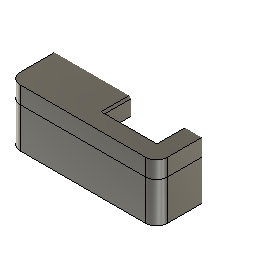
Password_key_ProMicro v1 (Autodesk Fusion 360 design; units mm, degrees)
Autodesk Fusion 360 part; units mm, degrees
sketch "Sketch1" plane through (0, 0, 0) normal (0, 0, 1) x (1, 0, 0)
  line L0 (0, 0) -> (33.5, 0)
  line L1 (33.5, 0) -> (33.5, 18.2)
  line L2 (33.5, 18.2) -> (0, 18.2)
  line L3 (0, 18.2) -> (0, 0)
  line L4 (-3, -3) -> (36.5, -3)
  line L5 (36.5, -3) -> (36.5, 21.2)
  line L6 (36.5, 21.2) -> (-3, 21.2)
  line L7 (-3, 21.2) -> (-3, -3)
  line L8 (0, 9.1) -> (-3, 9.1)
  line L9 (0, 12.85) -> (-3, 12.85)
  line L10 (-3, 12.85) -> (-3, 5.35)
  line L11 (-3, 5.35) -> (0, 5.35)
  line L12 (0, 5.35) -> (0, 12.85)
  line L13 (0, 12.85) -> (-3, 5.35) construction
  line L14 (-3, 12.85) -> (0, 5.35) construction
  circle A0 centre (0, 18.2) radius 0.5
  circle A1 centre (33.5, 18.2) radius 0.5
  circle A2 centre (0, 0) radius 0.5
  circle A3 centre (33.5, 0) radius 0.5
  point P0 (-1.5, 9.1)
  dimension "d1" = 33.5
  dimension "d2" = 18.2
  dimension "d3" = 3
  dimension "d4" = 7.5
  dimension "d10" = 1
  dimension "d11" = 1
  constraint horizontal L0
  constraint vertical L1
  constraint horizontal L2
  constraint vertical L3
  constraint coincident L0.start L3.end
  constraint midpoint L3 L8.start
  constraint midpoint L7 L8.end
  constraint horizontal L9
  constraint perpendicular L9 L10
  constraint parallel L9 L11
  constraint parallel L10 L12
  constraint coincident L13 P0
  constraint coincident L14 P0
  constraint coincident L3 L9.start
  constraint midpoint L8 P0
  constraint coincident L2.end L3.start
  constraint coincident L1.end L2.start
  constraint symmetric L8 A0 A2
  constraint symmetric L8 A1 A3
  measures "d1" distance of L0.start L0.end
  measures "d2" distance of L0.start L2.end
  measures "d4" distance of L9 L11
  measures "d10" diameter of A0
  measures "d11" diameter of A1
extrude "Extrude1" add sketch "Sketch1" against normal blind 1.75 contours L0 L1 L2 L3 L4 L5 L6 L7 L9 L11 A0 A1 A2 A3 makes body 1
extrude "Extrude2" add sketch "Sketch1" against normal blind 3 from surface at -1.75 bodies 1
fillet "Fillet1" radius 3 4 edges at (-3, -3, -2.375) (-3, 21.2, -2.375) (36.5, -3, -2.375) (36.5, 21.2, -2.375) on bodies 1
sketch "Sketch2" plane through (0, 0, 0) normal (0, 0, 1) x (1, 0, 0)
  line L0 (-3, 18.2) -> (-3, 12.85)
  line L1 (0, -3) -> (33.5, -3)
  line L2 (36.5, 0) -> (36.5, 18.2)
  line L3 (33.5, 21.2) -> (0, 21.2)
  line L4 (-3, 12.85) -> (0, 12.85)
  line L5 (0, 12.85) -> (0, 17.7)
  arc A0 (0.5, 18.2) -> (0, 17.7) centre (0, 18.2) ccw
  line L6 (0.5, 18.2) -> (33, 18.2)
  arc A1 (33.5, 17.7) -> (33, 18.2) centre (33.5, 18.2) ccw
  line L7 (33.5, 17.7) -> (33.5, 0.5)
  arc A2 (33, 0) -> (33.5, 0.5) centre (33.5, 0) ccw
  line L8 (33, 0) -> (0.5, 0)
  arc A3 (0, 0.5) -> (0.5, 0) centre (0, 0) ccw
  line L9 (0, 0.5) -> (0, 5.35)
  line L10 (0, 5.35) -> (-3, 5.35)
  arc A4 (36.5, 18.2) -> (33.5, 21.2) centre (33.5, 18.2) ccw
  arc A5 (0, 21.2) -> (-3, 18.2) centre (0, 18.2) ccw
  line L11 (-3, 5.35) -> (-3, 0)
  arc A6 (-3, 0) -> (0, -3) centre (0, 0) ccw
  arc A7 (33.5, -3) -> (36.5, 0) centre (33.5, 0) ccw
  line L12 (-1.4, 5.35) -> (-1.4, 0)
  arc A8 (-1.4, 0) -> (0, -1.4) centre (0, 0) ccw
  line L13 (0, -1.4) -> (33.5, -1.4)
  arc A9 (33.5, -1.4) -> (34.9, 0) centre (33.5, 0) ccw
  line L14 (34.9, 0) -> (34.9, 18.2)
  arc A10 (34.9, 18.2) -> (33.5, 19.6) centre (33.5, 18.2) ccw
  line L15 (33.5, 19.6) -> (0, 19.6)
  arc A11 (0, 19.6) -> (-1.4, 18.2) centre (0, 18.2) ccw
  line L16 (-1.4, 18.2) -> (-1.4, 12.85)
  dimension "d14" = -1.6
extrude "Extrude3" add sketch "Sketch2" along normal blind 6 contours L0 L1 L2 L3 L4 L10 A4 A5 L11 A6 A7 L12 A8 L13 A9 L14 A10 L15 A11 L16 bodies 1
sketch "Sketch3" plane through (0, 0, 6) normal (0, 0, 1) x (-1, 0, 0)
  line L0 (1.4, -5.35) -> (3, -5.35)
  line L1 (3, -5.35) -> (3, 0)
  arc A0 (3, 0) -> (0, 3) centre (0, 0) ccw
  line L2 (0, 3) -> (-33.5, 3)
  arc A1 (-33.5, 3) -> (-36.5, 0) centre (-33.5, 0) ccw
  line L3 (-36.5, 0) -> (-36.5, -18.2)
  arc A2 (-36.5, -18.2) -> (-33.5, -21.2) centre (-33.5, -18.2) ccw
  line L4 (-33.5, -21.2) -> (0, -21.2)
  arc A3 (0, -21.2) -> (3, -18.2) centre (0, -18.2) ccw
  line L5 (3, -18.2) -> (3, -12.85)
  line L6 (3, -12.85) -> (1.4, -12.85)
  line L7 (1.4, -12.85) -> (1.4, -18.2)
  arc A4 (0, -19.6) -> (1.4, -18.2) centre (0, -18.2) ccw
  line L8 (0, -19.6) -> (-33.5, -19.6)
  arc A5 (-34.9, -18.2) -> (-33.5, -19.6) centre (-33.5, -18.2) ccw
  line L9 (-34.9, -18.2) -> (-34.9, 0)
  arc A6 (-33.5, 1.4) -> (-34.9, 0) centre (-33.5, 0) ccw
  line L10 (-33.5, 1.4) -> (0, 1.4)
  arc A7 (1.4, 0) -> (0, 1.4) centre (0, 0) ccw
  line L11 (1.4, 0) -> (1.4, -5.35)
  arc A8 (-36.5, -18.2) -> (-33.5, -21.2) centre (-33.5, -18.2) ccw
  line L12 (-36.5, -18.2) -> (-36.5, 0)
  arc A9 (-33.5, 3) -> (-36.5, 0) centre (-33.5, 0) ccw
  line L13 (-33.5, 3) -> (0, 3)
  arc A10 (3, 0) -> (0, 3) centre (0, 0) ccw
  line L14 (3, 0) -> (3, -18.2)
  arc A11 (0, -21.2) -> (3, -18.2) centre (0, -18.2) ccw
  line L15 (0, -21.2) -> (-33.5, -21.2)
extrude "Extrude4" add sketch "Sketch3" 1 faces at (11.1667, -1.9333, 6) along normal blind 1.6 separate body contours L0 L6 L7 A4 L8 A5 L9 A6 L10 A7 L11 L14 on bodies 1 makes body 2
sketch "Sketch4" plane through (0, 0, 6) normal (0, 0, -1) x (1, 0, 0)
  line L0 (-3, 0) -> (-3, -18.2)
  arc A0 (-3, -18.2) -> (0, -21.2) centre (0, -18.2) ccw
  line L1 (0, -21.2) -> (33.5, -21.2)
  arc A1 (33.5, -21.2) -> (36.5, -18.2) centre (33.5, -18.2) ccw
  line L2 (36.5, -18.2) -> (36.5, 0)
  arc A2 (36.5, 0) -> (33.5, 3) centre (33.5, 0) ccw
  line L3 (33.5, 3) -> (0, 3)
  arc A3 (0, 3) -> (-3, 0) centre (0, 0) ccw
  line L4 (-3, -5.35) -> (0, -5.35)
  line L5 (0, -12.85) -> (-3, -12.85)
  line L6 (-3, -21.2) -> (-3, 3)
  line L7 (0, -5.35) -> (0, -12.85)
  line L8 (-3, -5.45) -> (0, -5.45)
  line L9 (-3, -9.1) -> (0, -9.1)
  line L10 (-3, -12.75) -> (0, -12.75)
  dimension "d19" = 0.1
  constraint midpoint L6 L9.start
  constraint midpoint L7 L9.end
  constraint symmetric L8.start L9 L10.start
  constraint symmetric L8.end L9 L10.end
extrude "Extrude5" add sketch "Sketch4" along normal blind 3 contours L0 L6 L7 L8 L9 | L0 L6 L7 L9 L10 bodies 2
sketch "Sketch5" plane through (0, 0, 6) normal (0, 0, -1) x (1, 0, 0)
  line L0 (0, -12.75) -> (-3, -12.75)
  line L1 (-3, -12.75) -> (-3, -18.2)
  arc A0 (-3, -18.2) -> (0, -21.2) centre (0, -18.2) ccw
  line L2 (0, -21.2) -> (33.5, -21.2)
  arc A1 (33.5, -21.2) -> (36.5, -18.2) centre (33.5, -18.2) ccw
  line L3 (36.5, -18.2) -> (36.5, 0)
  arc A2 (36.5, 0) -> (33.5, 3) centre (33.5, 0) ccw
  line L4 (33.5, 3) -> (0, 3)
  arc A3 (0, 3) -> (-3, 0) centre (0, 0) ccw
  line L5 (-3, 0) -> (-3, -5.45)
  line L6 (-3, -5.45) -> (0, -5.45)
  line L7 (0, -5.45) -> (0, -12.75)
  line L8 (-1.4, -5.35) -> (-3, -5.35)
  line L9 (-3, -5.35) -> (-3, 0)
  arc A4 (0, 3) -> (-3, 0) centre (0, 0) ccw
  line L10 (0, 3) -> (33.5, 3)
  arc A5 (36.5, 0) -> (33.5, 3) centre (33.5, 0) ccw
  line L11 (36.5, 0) -> (36.5, -18.2)
  arc A6 (33.5, -21.2) -> (36.5, -18.2) centre (33.5, -18.2) ccw
  line L12 (33.5, -21.2) -> (0, -21.2)
  arc A7 (-3, -18.2) -> (0, -21.2) centre (0, -18.2) ccw
  line L13 (-3, -18.2) -> (-3, -12.85)
  line L14 (-3, -12.85) -> (-1.4, -12.85)
  line L15 (-1.4, -12.85) -> (-1.4, -18.2)
  arc A8 (-1.4, -18.2) -> (0, -19.6) centre (0, -18.2) ccw
  line L16 (0, -19.6) -> (33.5, -19.6)
  arc A9 (33.5, -19.6) -> (34.9, -18.2) centre (33.5, -18.2) ccw
  line L17 (34.9, -18.2) -> (34.9, 0)
  arc A10 (34.9, 0) -> (33.5, 1.4) centre (33.5, 0) ccw
  line L18 (33.5, 1.4) -> (0, 1.4)
  arc A11 (0, 1.4) -> (-1.4, 0) centre (0, 0) ccw
  line L19 (-1.4, 0) -> (-1.4, -5.35)
  line L20 (-1.2, -12.85) -> (-1.2, -18.2)
  arc A12 (-1.2, -18.2) -> (0, -19.4) centre (0, -18.2) ccw
  line L21 (0, -19.4) -> (33.5, -19.4)
  arc A13 (33.5, -19.4) -> (34.7, -18.2) centre (33.5, -18.2) ccw
  line L22 (34.7, -18.2) -> (34.7, 0)
  arc A14 (34.7, 0) -> (33.5, 1.2) centre (33.5, 0) ccw
  line L23 (33.5, 1.2) -> (0, 1.2)
  arc A15 (0, 1.2) -> (-1.2, 0) centre (0, 0) ccw
  line L24 (-1.2, 0) -> (-1.2, -5.35)
  line L25 (-1.2, -12.85) -> (-1.2, -12.75)
  line L26 (-1.2, -12.75) -> (-1.2, -5.35)
  line L27 (0.4, -12.85) -> (0.4, -17.8)
  line L28 (0.4, -17.8) -> (33.1, -17.8)
  line L29 (33.1, -17.8) -> (33.1, -0.4)
  line L30 (33.1, -0.4) -> (0.4, -0.4)
  line L31 (0.4, -0.4) -> (0.4, -5.35)
  line L32 (0.4, -12.85) -> (0.4, -5.35)
  dimension "d22" = -0.2
  dimension "d23" = -1.8
  constraint coincident L0 L25.end
  constraint perpendicular L0 L25
  constraint perpendicular L8 L26
extrude "Extrude6" add sketch "Sketch5" along normal blind 3 contours L0 L6 L7 L20 A12 L21 A13 L22 A14 L23 A15 L24 L25 L26 bodies 2
sketch "Sketch6" plane through (0, 0, 7.6) normal (0, 0, 1) x (-1, 0, 0)
  line L0 (3, -18.2) -> (3, 0)
  arc A0 (3, 0) -> (0, 3) centre (0, 0) ccw
  line L1 (0, 3) -> (-33.5, 3)
  arc A1 (-33.5, 3) -> (-36.5, 0) centre (-33.5, 0) ccw
  line L2 (-36.5, 0) -> (-36.5, -18.2)
  arc A2 (-36.5, -18.2) -> (-33.5, -21.2) centre (-33.5, -18.2) ccw
  line L3 (-33.5, -21.2) -> (0, -21.2)
  arc A3 (0, -21.2) -> (3, -18.2) centre (0, -18.2) ccw
  line L4 (3, -9.1) -> (-36.5, -9.1)
  line L5 (-31.5, -16.09) -> (-17.52, -16.09)
  line L6 (-17.52, -16.09) -> (-17.52, -2.11)
  line L7 (-17.52, -2.11) -> (-31.5, -2.11)
  line L8 (-31.5, -2.11) -> (-31.5, -16.09)
  line L9 (-31.5, -16.09) -> (-17.52, -2.11) construction
  line L10 (-17.52, -16.09) -> (-31.5, -2.11) construction
  point P0 (-24.51, -9.1)
  dimension "d26" = 13.98
  dimension "d27" = 13.98
  dimension "d28" = 5
  constraint midpoint L0 L4.start
  constraint midpoint L2 L4.end
  constraint horizontal L5
  constraint perpendicular L5 L6
  constraint parallel L5 L7
  constraint parallel L6 L8
  constraint coincident L9 P0
  constraint coincident L10 P0
  constraint coincident L4 P0
  measures "d26" distance of L6.end L7.end
  measures "d27" distance of L5.end L6.end
  measures "d28" distance of L2 L8
extrude "Extrude7" add sketch "Sketch6" along normal blind 3 contours L0 L2 A2 L3 A3 L4 L5 L6 L8 | L0 A0 L1 A1 L2 L4 L6 L7 L8 bodies 2
extrude "Extrude8" cut 1 faces at (26.84, 6.77, 7.6) along direction (0, 0, -1) blind 2.947 on bodies 2 bodies 2
sketch "Sketch7" plane through (0, -1.2, 0) normal (0, -1, 0) x (1, 0, 0)
  line L0 (33.5, 6) -> (0, 6)
  line L1 (0, 6) -> (0, 3)
  line L2 (0, 3) -> (33.5, 3)
  line L3 (33.5, 3) -> (33.5, 6)
  line L4 (14.25, 3.4) -> (19.25, 3.4)
  line L5 (19.25, 3.4) -> (19.25, 5.2)
  line L6 (19.25, 5.2) -> (14.25, 5.2)
  line L7 (14.25, 5.2) -> (14.25, 3.4)
  line L8 (14.05, 3.2) -> (19.45, 3.2)
  line L9 (19.45, 3.2) -> (19.45, 5.4)
  line L10 (19.45, 5.4) -> (14.05, 5.4)
  line L11 (14.05, 5.4) -> (14.05, 3.2)
  line L12 (16.75, 3) -> (16.75, 6)
  line L13 (33.5, 6) -> (0, 6)
  point P0 (16.75, 5.4)
  dimension "d33" = 5
  dimension "d34" = 1.8
  dimension "d35" = 0.2
  dimension "d42" = 0.6
  constraint horizontal L4
  constraint vertical L5
  constraint horizontal L6
  constraint vertical L7
  constraint midpoint L2 L12.start
  constraint midpoint L0 L12.end
  constraint midpoint L10 P0
  constraint coincident L12 P0
  measures "d33" distance of L4.start L4.end
  measures "d34" distance of L4.start L6.end
  measures "d42" distance of L10 L13
extrude "Extrude9" add sketch "Sketch7" along normal blind 10 draft -45 contours L4 L6 L7 L12 | L4 L5 L6 L12 bodies 2
extrude "Extrude10" cut sketch "Sketch7" along normal blind 15 draft -45 from surface at 0.2 contours L4 L6 L7 L8 L10 L11 L12 | L4 L5 L6 L8 L9 L10 L12 | L4 L6 L7 L12 | L4 L5 L6 L12 bodies 1
ref_plane "WorkPlane1" through (16.75, 9.1, 0.625) normal (0, 1, 0) x (1, 0, 0)
mirror "Mirror1" about plane through (16.75, 9.1, 0.625) normal (0, 1, 0) of "Extrude9", "Extrude10"
sketch "Sketch8" plane through (34.7, 0, 0) normal (1, 0, 0) x (0, 1, 0)
  line L0 (18.2, 6) -> (0, 6)
  line L1 (0, 6) -> (0, 3)
  line L2 (0, 3) -> (18.2, 3)
  line L3 (18.2, 3) -> (18.2, 6)
  line L4 (9.1, 6) -> (9.1, 3)
  line L5 (11.6, 3.6) -> (6.6, 3.6)
  line L6 (6.6, 3.6) -> (6.6, 5.4)
  line L7 (6.6, 5.4) -> (11.6, 5.4)
  line L8 (11.6, 5.4) -> (11.6, 3.6)
  line L9 (11.6, 3.6) -> (6.6, 5.4) construction
  line L10 (6.6, 3.6) -> (11.6, 5.4) construction
  line L11 (0, 6) -> (18.2, 6)
  line L12 (11.8, 3.4) -> (6.4, 3.4)
  line L13 (6.4, 3.4) -> (6.4, 5.6)
  line L14 (6.4, 5.6) -> (11.8, 5.6)
  line L15 (11.8, 5.6) -> (11.8, 3.4)
  point P0 (9.1, 4.5)
  dimension "d45" = 5
  dimension "d46" = 1.8
  dimension "d48" = -0.2
  dimension "d49" = 0.4
  constraint midpoint L0 L4.start
  constraint midpoint L2 L4.end
  constraint horizontal L5
  constraint perpendicular L5 L6
  constraint parallel L5 L7
  constraint parallel L6 L8
  constraint coincident L9 P0
  constraint coincident L10 P0
  constraint coincident L4 P0
  measures "d45" distance of L6.end L7.end
  measures "d46" distance of L5.end L6.end
  measures "d49" distance of L11 L14
extrude "Extrude11" add sketch "Sketch8" along normal blind 15 draft -45 contours L4 L5 L7 L8 | L4 L5 L6 L7 bodies 2
extrude "Extrude12" cut sketch "Sketch8" along normal blind 1.8 draft -45 from surface at 0.2 contours L4 L5 L7 L8 L12 L14 L15 | L4 L5 L6 L7 L12 L13 L14 | L4 L5 L7 L8 | L4 L5 L6 L7 bodies 1
fillet "Fillet2" radius 0.4 3 edges at (35.6, 9.1, 4.5) (16.75, -2.1, 4.3) (16.75, 20.3, 4.3) on bodies 2
chamfer "Chamfer1" distance 0.4 angle 45 9 edges at (16.75, 19.4, 3) (34.3485, 19.0485, 3) (34.7, 9.1, 3) (34.3485, -0.8485, 3) (16.75, -1.2, 3) (-0.8485, -0.8485, 3) (-1.2, 2.725, 3) (-1.2, 15.475, 3) (-0.8485, 19.0485, 3) on bodies 2
chamfer "Chamfer2" distance 0.5 angle 45 4 edges at (17.52, 9.1, 10.6) (24.51, 16.09, 10.6) (31.5, 9.1, 10.6) (24.51, 2.11, 10.6) on bodies 2
named bodies: "Base", "Cover"
